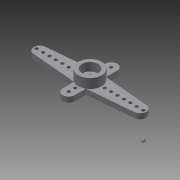
# Autodesk Inventor part: servo micro arm
Saved by Autodesk Inventor 2015 SP2 (Build 190223200, 223)
## iProperties
Created: 2015-05-24
Part Number: servo micro arm
Material: Generic
Document SubType Name: Modeling
Designer: caleb
Density: 1 g/cm^3
Appearance: Default
Author: caleb
Autodesk Inventor part; units mm, degrees
ref_plane "YZ Plane" through (0, 0, 0) normal (1, 0, 0) x (0, 1, 0)
ref_plane "XZ Plane" through (0, 0, 0) normal (0, 1, 0) x (-1, 0, 0)
sketch "Sketch1" plane through (0, 0, 0) normal (0, 0, 1) x (1, 0, 0)
  circle A0 centre (0, 0) radius 3.55
  line L0 (-1.82, -3.048) -> (-1.82, -6.48)
  arc A1 (-1.82, -6.48) -> (1.82, -6.48) centre (0, -6.48) ccw
  line L1 (1.82, -6.48) -> (1.82, -3.048)
  line L2 (0, -6.48) -> (0, -8.3) construction
  line L3 (0, -6.48) -> (0, -3.55) construction
  line L4 (1.82, -3.048) -> (15.3644, -1.8326)
  arc A2 (15.3644, -1.8326) -> (15.3644, 1.8326) centre (15.2, 0) ccw
  line L5 (15.3644, 1.8326) -> (1.82, 3.048)
  line L6 (1.82, 3.048) -> (1.82, 6.48)
  arc A3 (1.82, 6.48) -> (-1.82, 6.48) centre (0, 6.48) ccw
  line L7 (-1.82, 6.48) -> (-1.82, 3.048)
  line L8 (-1.82, 3.048) -> (-15.3644, 1.8326)
  arc A4 (-15.3644, 1.8326) -> (-15.3644, -1.8326) centre (-15.2, 0) ccw
  line L9 (-15.3644, -1.8326) -> (-1.82, -3.048)
  line L10 (-17.04, 0) -> (17.04, 0) construction
  dimension "d0" = 7.1
  dimension "d1" = 3.64
  dimension "d2" = 8.3
  dimension "d3" = 34.08
  dimension "d4" = 1.84
  constraints: 22 end point, 16 point on circle, 8 tangent, 5 centre point, 3 horizontal alignment, 2 collinear, 2 equal length, 2 parallel, 2 vertical, 1 coincident, 1 equal radius, 1 horizontal, 1 point on line, 1 vertical alignment
  measures "d0" diameter of A0
  measures "d1" distance between parallel lines of L0 L1
  measures "d2" distance of L2.end point (0, 0)
  measures "d3" distance of L10.start L10.end
  measures "d4" radius of A4
extrude "Extrusion1" add sketch "Sketch1" against normal blind 1.57
extrude "Extrusion2" add sketch "Sketch1" along normal blind 2.87 contours A0
sketch "Sketch2" plane through (0, 0, 2.87) normal (0, 0, 1) x (1, 0, 0)
  circle A0 centre (0, 0) radius 2.435
  circle A1 centre (0, 0) radius 1.25
  dimension "d9" = 4.87
  dimension "d10" = 2.5
  constraints: 2 centre point, 2 coincident
  measures "d9" diameter of A0
  measures "d10" diameter of A1
extrude "Extrusion3" cut sketch "Sketch2" against normal blind 2.5 contours A0 | A1
extrude "Extrusion4" cut sketch "Sketch2" against normal through all contours A1
sketch "Sketch3" plane through (0, 0, -1.57) normal (0, 0, -1) x (-1, 0, 0)
  circle A0 centre (0, 0) radius 2.475
  dimension "d15" = 4.95
  constraints: 1 centre point, 1 coincident
  measures "d15" diameter of A0
extrude "Extrusion5" cut sketch "Sketch3" against normal blind 1
sketch "Sketch4" plane through (0, 0, -1.57) normal (0, 0, -1) x (-1, 0, 0)
  circle A0 centre (0, 0) radius 2.475 construction
  line L0 (1.82, -6.48) -> (1.82, -3.048) construction
  line L1 (1.82, -3.048) -> (15.3644, -1.8326) construction
  arc A1 (15.3644, -1.8326) -> (15.3644, 1.8326) centre (15.2, 0) ccw construction
  line L2 (15.3644, 1.8326) -> (1.82, 3.048) construction
  line L3 (1.82, 3.048) -> (1.82, 6.48) construction
  arc A2 (1.82, 6.48) -> (-1.82, 6.48) centre (0, 6.48) ccw construction
  line L4 (-1.82, 6.48) -> (-1.82, 3.048) construction
  line L5 (-1.82, 3.048) -> (-15.3644, 1.8326) construction
  arc A3 (-15.3644, 1.8326) -> (-15.3644, -1.8326) centre (-15.2, 0) ccw construction
  line L6 (-15.3644, -1.8326) -> (-1.82, -3.048) construction
  line L7 (-1.82, -3.048) -> (-1.82, -6.48) construction
  arc A4 (-1.82, -6.48) -> (1.82, -6.48) centre (0, -6.48) ccw construction
  circle A5 centre (4.475, 0) radius 0.5
  circle A6 centre (0, -4.475) radius 0.5
  dimension "d18" = 1
  dimension "d19" = 4.475
  dimension "d20" = 4.475
  constraints: 2 centre point, 1 equal radius, 1 horizontal alignment, 1 vertical alignment
  measures "d18" diameter of A5
  measures "d19" distance of point (0, 0) A5.centre
  measures "d20" distance of A6.centre point (0, 0)
extrude "Extrusion6" cut sketch "Sketch4" against normal through all contours A5
pattern_linear "Rectangular Pattern1" count 7 spacing 1.95 along (-1, 0, 0) of "Extrusion6"
pattern_circular "Circular Pattern1" count 2 over 360 about axis through (0, 0, -10) along (0, 0, 1) of "Extrusion6", "Rectangular Pattern1"
extrude "Extrusion7" cut sketch "Sketch4" against normal through all contours A6
pattern_linear "Rectangular Pattern2" count 2 spacing 1.95 along (0, -1, 0) of "Extrusion7"
pattern_circular "Circular Pattern2" count 2 over 360 about axis through (0, 0, -10) along (0, 0, 1) of "Extrusion7", "Rectangular Pattern2"
ref_plane "Work Plane1" through (0, 0, -7.92) normal (0, 0, -1) x (-1, 0, 0)
sketch "Sketch5" plane through (0, 0, -7.92) normal (0, 0, -1) x (-1, 0, 0)
  circle A0 centre (-16.175, 0) radius 0.5 construction
  arc A1 (-16.175, -0.5) -> (-16.175, 0.5) centre (-16.175, 0) ccw
  line L0 (-16.175, 0.5) -> (-16.175, -0.5)
  constraints: 3 coincident, 2 end point, 2 point on circle, 1 centre point, 1 concentric, 1 midpoint, 1 vertical
revolve "Revolution1" add sketch "Sketch5" angle 360 about axis through (16.175, 0.5, -7.92) along (0, -1, 0) separate body
equation "\"d20\" = d19"
body "Solid1"
body "Solid2"
